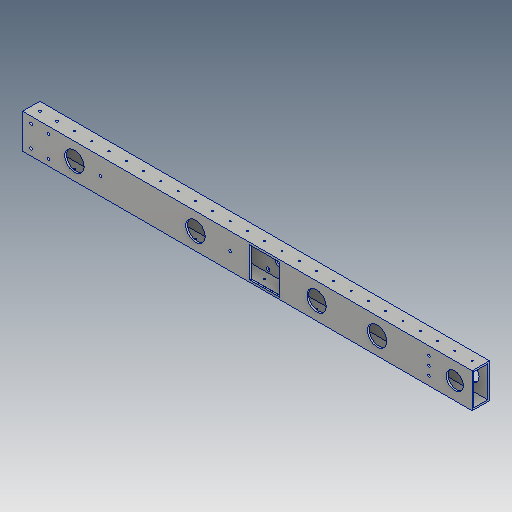
# Autodesk Inventor part: Vert Uprights
Saved by Autodesk Inventor 2018 (Build 220112000, 112)
## iProperties
Created: 2018-01-08
Part Number: Vert Uprights
Material: Aluminum 6061
Document SubType Name: Modeling
Designer: dsayers
Density: 2.7 g/cm^3
Appearance: Aluminum - Flat
Mass: 573.49 g
Surface Area: 1700.04 cm^2
Volume: 212.404 cm^3
Author: dsayers
Autodesk Inventor part; units mm, degrees
ref_plane "YZ Plane" through (0, 0, 0) normal (1, 0, 0) x (0, 1, 0)
ref_plane "XZ Plane" through (0, 0, 0) normal (0, 1, 0) x (-1, 0, 0)
ref_plane "XY Plane" through (0, 0, 0) normal (0, 0, 1) x (1, 0, 0)
sketch "Sketch1" plane through (0, 0, 0) normal (0, 0, 1) x (1, 0, 0)
  line L0 (0, 0) -> (25.4, 0)
  line L1 (25.4, 0) -> (25.4, 50.8)
  line L2 (25.4, 50.8) -> (0, 50.8)
  line L3 (0, 50.8) -> (0, 0)
  dimension "d0" = 25.4
  dimension "d1" = 50.8
  constraints: 8 end point, 2 parallel, 1 horizontal, 1 perpendicular
  measures "d0" distance of L1.end L2.end
  measures "d1" distance of L0.end L1.end
extrude "Extrusion1" add sketch "Sketch1" along normal blind 609.6
shell "Shell1" thickness 2.54 removed faces 2 at (8.4667, 33.8667, 0) at (8.4667, 33.8667, 609.6)
sketch "Sketch2" plane through (0, 50.8, 0) normal (0, 1, 0) x (1, 0, 0)
  line L0 (25.4, 0) -> (0, 0) projected
  line L1 (0, 0) -> (0, -609.6) projected
  point P0 (12.7, -12.7)
  point P1 (12.7, -38.1)
  point P2 (12.7, -63.5)
  point P3 (12.7, -88.9)
  point P4 (12.7, -114.3)
  point P5 (12.7, -139.7)
  point P6 (12.7, -165.1)
  point P7 (12.7, -190.5)
  point P8 (12.7, -215.9)
  point P9 (12.7, -241.3)
  point P10 (12.7, -266.7)
  point P11 (12.7, -292.1)
  point P12 (12.7, -317.5)
  point P13 (12.7, -342.9)
  point P14 (12.7, -368.3)
  point P15 (12.7, -393.7)
  point P16 (12.7, -419.1)
  point P17 (12.7, -444.5)
  point P18 (12.7, -469.9)
  point P19 (12.7, -495.3)
  point P20 (12.7, -520.7)
  point P21 (12.7, -546.1)
  point P22 (12.7, -571.5)
  point P23 (12.7, -596.9)
  point P24 (12.7, -622.3)
  point P25 (12.7, -647.7)
  point P26 (12.7, -673.1)
  point P27 (12.7, -698.5)
  point P28 (12.7, -723.9)
  point P29 (12.7, -749.3)
  point P30 (12.7, -774.7)
  point P31 (12.7, -800.1)
  point P32 (12.7, -825.5)
  point P33 (12.7, -850.9)
  point P34 (12.7, -876.3)
  point P35 (12.7, -901.7)
  point P36 (12.7, -927.1)
  dimension "d5" = 12.7
  dimension "d6" = 12.7
  dimension "d9" = 25.4
  constraints: 1 vertical, 36 other
  measures "d5" distance from line of L0 point (12.7, -12.7)
  measures "d6" distance from line of L1 point (12.7, -12.7)
  measures "d9" distance of point (12.7, -12.7) point (12.7, -38.1)
hole "Hole1" at (12.7, 50.8, 12.7) at (12.7, 50.8, 38.1) at (12.7, 50.8, 63.5) at (12.7, 50.8, 88.9) at (12.7, 50.8, 114.3) at (12.7, 50.8, 139.7) at (12.7, 50.8, 165.1) at (12.7, 50.8, 190.5) at (12.7, 50.8, 215.9) at (12.7, 50.8, 241.3) at (12.7, 50.8, 266.7) at (12.7, 50.8, 292.1) at (12.7, 50.8, 317.5) at (12.7, 50.8, 342.9) at (12.7, 50.8, 368.3) at (12.7, 50.8, 393.7) at (12.7, 50.8, 419.1) at (12.7, 50.8, 444.5) at (12.7, 50.8, 469.9) at (12.7, 50.8, 495.3) at (12.7, 50.8, 520.7) at (12.7, 50.8, 546.1) at (12.7, 50.8, 571.5) at (12.7, 50.8, 596.9) at (12.7, 50.8, 622.3) at (12.7, 50.8, 647.7) at (12.7, 50.8, 673.1) at (12.7, 50.8, 698.5) at (12.7, 50.8, 723.9) at (12.7, 50.8, 749.3) at (12.7, 50.8, 774.7) at (12.7, 50.8, 800.1) at (12.7, 50.8, 825.5) at (12.7, 50.8, 850.9) at (12.7, 50.8, 876.3) at (12.7, 50.8, 901.7) direction (0, -1, 0) diameter 2.54 depth 50.8 tip angle 118
sketch "Sketch6" plane through (0, 0, 0) normal (-1, 0, 0) x (0, 0, 1)
  line L0 (0, 50.8) -> (0, 0) projected
  line L1 (0, 0) -> (609.6, 0) projected
  point P0 (304.8, 25.4)
  dimension "d48" = 304.8
  dimension "d49" = 25.4
  measures "d48" distance from line of L0 point (304.8, 25.4)
  measures "d49" distance from line of L1 point (304.8, 25.4)
hole "Hole5" at (0, 25.4, 304.8) direction (1, 0, 0) diameter 15.875 depth 25.4 tip angle 118
sketch "Sketch7" plane through (25.4, 0, 0) normal (1, 0, 0) x (0, 0, -1)
  line L0 (0, 50.8) -> (-609.6, 50.8) projected
  circle A0 centre (-304.8, 25.4) radius 7.9375 projected
  point P0 (0, 0)
  point P1 (-584.2, 25.4)
  dimension "d57" = 25.4
  dimension "d58" = 279.4
  measures "d57" distance from line of L0 point (-584.2, 25.4)
  measures "d58" distance of A0.centre point (-584.2, 25.4)
hole "Hole6" at (25.4, 25.4, 584.2) direction (-1, 0, 0) diameter 25.4 depth 25.4 tip angle 118
sketch "Sketch8" plane through (0, 0, 0) normal (-1, 0, 0) x (0, 0, 1)
  circle A0 centre (304.8, 25.4) radius 7.9375 projected
  line L0 (282.575, 47.625) -> (327.025, 47.625)
  line L1 (327.025, 47.625) -> (327.025, 3.175)
  line L2 (327.025, 3.175) -> (282.575, 3.175)
  line L3 (282.575, 3.175) -> (282.575, 47.625)
  line L4 (282.575, 47.625) -> (327.025, 3.175) construction
  line L5 (327.025, 47.625) -> (282.575, 3.175) construction
  point P0 (0, 0)
  dimension "d66" = 44.45
  dimension "d67" = 44.45
  constraints: 12 end point, 2 midpoint, 2 parallel, 1 horizontal, 1 perpendicular
  measures "d66" distance of L0.end L1.end
  measures "d67" distance of L1.end L2.end
extrude "Extrusion2" cut sketch "Sketch8" against normal blind 12.7 contours A0 | L0 L1 L2 L3
sketch "Sketch9" plane through (25.4, 0, 0) normal (1, 0, 0) x (0, 0, -1)
  arc A0 (-320.6117, 44.0059) -> (-323.0807, 41.5866) centre (-322.5771, 43.5421) ccw projected
  arc A1 (-288.9883, 6.7941) -> (-286.5193, 9.2134) centre (-287.0229, 7.2579) ccw projected
  circle A2 centre (-322.4769, 8.0788) radius 3.3655 projected
  circle A3 centre (-287.1231, 42.7212) radius 3.1115 projected
  point P0 (0, 0)
  constraints: 4 coincident
hole "Hole7" at (25.4, 8.0788, 322.4769) at (25.4, 43.5421, 322.5771) at (25.4, 42.7212, 287.1231) at (25.4, 7.2579, 287.0229) direction (-1, 0, 0) diameter 5.6134 depth 25.4 tip angle 118 clearance for "Flat Head Machine Screw (82)" size "#10" standard "Ansi Unified Screw Threads"
sketch "Sketch10" plane through (0, 0, 0) normal (0, 0, -1) x (-1, 0, 0)
  line L0 (-2.54, 48.26) -> (-2.54, 2.54) projected
  line L1 (-2.54, 2.54) -> (-22.86, 2.54) projected
  line L2 (-22.86, 2.54) -> (-22.86, 48.26) projected
  line L3 (-22.86, 48.26) -> (-2.54, 48.26) projected
  line L4 (0, 0) -> (-25.4, 0) projected
  line L5 (0, 50.8) -> (0, 0) projected
  line L6 (-25.4, 50.8) -> (0, 50.8) projected
  line L7 (-25.4, 0) -> (-25.4, 50.8) projected
extrude "Extrusion3" add sketch "Sketch10" along normal blind 50.8
sketch "Sketch11" plane through (0, 50.8, 609.6) normal (0, 1, 0) x (1, 0, 0)
  circle A0 centre (12.7, 596.9) radius 1.27 projected
  line L0 (25.4, 660.4) -> (25.4, 0) projected
  point P0 (0, 609.6)
  point P1 (12.7, 622.3)
  point P2 (12.7, 647.7)
  dimension "d79" = 25.4
  dimension "d80" = 25.4
  dimension "d81" = 12.7
  dimension "d82" = 12.7
  measures "d79" distance of point (12.7, 622.3) point (12.7, 647.7)
  measures "d80" distance of A0.centre point (12.7, 622.3)
  measures "d81" distance from line of L0 point (12.7, 622.3)
  measures "d82" distance from line of L0 point (12.7, 647.7)
hole "Hole8" at (12.7, 50.8, -12.7) at (12.7, 50.8, -38.1) direction (0, -1, 0) diameter 3.9116 depth 50.8 tip angle 118 clearance for "Flat Head Machine Screw (82)" size "#5" standard "Ansi Unified Screw Threads"
sketch "Sketch12" plane through (0, 0, 609.6) normal (-1, 0, 0) x (0, 0, 1)
  circle A0 centre (-63.5, 25.4) radius 1.27 projected
  line L0 (0, 0) -> (-660.4, 0) projected
  line L1 (-660.4, 50.8) -> (0, 50.8) projected
  point P0 (-609.6, 0)
  point P1 (-63.5, 38.1)
  point P2 (-63.5, 12.7)
  dimension "d90" = 12.7
  dimension "d91" = 12.7
  dimension "d106" = 0
  dimension "d107" = 0
  constraints: 1 coincident
  measures "d90" distance from line of L0 point (-63.5, 12.7)
  measures "d91" distance from line of L1 point (-63.5, 38.1)
  measures "d106" horizontal distance of point (-63.5, 12.7) A0.centre
  measures "d107" horizontal distance of point (-63.5, 38.1) A0.centre
hole "Hole9" at (0, 25.4, 546.1) at (0, 38.1, 546.1) at (0, 12.7, 546.1) direction (1, 0, 0) diameter 3.9116 depth 50.8 tip angle 118 clearance for "Flat Head Machine Screw (82)" size "#5" standard "Ansi Unified Screw Threads"
sketch "Sketch13" plane through (0, 0, 609.6) normal (-1, 0, 0) x (0, 0, 1)
  circle A0 centre (-622.3, 533.4) radius 2.8067 projected
  circle A1 centre (-647.7, 533.4) radius 2.8067 projected
  circle A2 centre (-622.3, 584.2) radius 2.8067 projected
  circle A3 centre (-647.7, 584.2) radius 2.8067 projected
  circle A4 centre (-635, 558.8) radius 2.8067 projected
  circle A5 centre (-635, 190.5) radius 2.8067 projected
  circle A6 centre (-635, 762) radius 2.8067 projected
  circle A7 centre (-622.3, 762) radius 2.8067 projected
  circle A8 centre (-622.3, 558.8) radius 2.8067 projected
  circle A9 centre (-622.3, 190.5) radius 2.8067 projected
  circle A10 centre (-647.7, 190.5) radius 2.8067 projected
  circle A11 centre (-647.7, 558.8) radius 2.8067 projected
  circle A12 centre (-647.7, 762) radius 2.8067 projected
  circle A13 centre (-647.7, 41.275) radius 2.8067 projected
  circle A14 centre (-622.3, 41.275) radius 2.8067 projected
  circle A15 centre (-647.7, 9.525) radius 2.8067 projected
  circle A16 centre (-622.3, 9.525) radius 2.8067 projected
  circle A17 centre (-635, 374.65) radius 14.2875 projected
  circle A18 centre (-635, 114.3) radius 14.2875 projected
  circle A19 centre (-635, 730.25) radius 6.35 projected
  circle A20 centre (-635, 615.95) radius 6.35 projected
  circle A21 centre (-635, 649.2875) radius 2.8067 projected
  circle A22 centre (-635, 696.9125) radius 2.8067 projected
  circle A23 centre (-635, 673.1) radius 19.05 projected
  line L0 (-609.6, 774.7) -> (-660.4, 774.7) projected
  line L1 (-660.4, 774.7) -> (-660.4, -25.4) projected
  line L2 (-609.6, -25.4) -> (-660.4, -25.4) projected
  line L3 (-609.6, 774.7) -> (-609.6, -25.4) projected
  point P0 (-609.6, 0)
  constraints: 4 coincident
hole "Hole10" at (0, 41.275, -12.7) at (0, 9.525, -12.7) at (0, 9.525, -38.1) at (0, 41.275, -38.1) direction (1, 0, 0) diameter 3.9116 depth 50.8 tip angle 118 clearance for "Flat Head Machine Screw (82)" size "#5" standard "Ansi Unified Screw Threads"
sketch "Sketch14" plane through (0, 0, 609.6) normal (-1, 0, 0) x (0, 0, 1)
  circle A0 centre (-139.7, 25.4) radius 14.2875
  line L0 (-76.2, 546.1) -> (-76.2, 0) projected
  line L1 (0, 0) -> (-660.4, 0) projected
  point P0 (-609.6, 0)
  dimension "d108" = 63.5
  dimension "d109" = 28.575
  dimension "d110" = 25.4
  constraints: 1 centre point
  measures "d108" distance from line of L0 A0.centre
  measures "d109" diameter of A0
  measures "d110" distance from line of L1 A0.centre
extrude "Extrusion4" cut sketch "Sketch14" against normal blind 50.8
sketch "Sketch15" plane through (0, 0, 609.6) normal (-1, 0, 0) x (0, 0, 1)
  line L0 (0, 0) -> (-660.4, 0) projected
  line L1 (-660.4, 0) -> (-660.4, 50.8) projected
  point P0 (-609.6, 0)
  point P1 (-355.6, 25.4)
  dimension "d113" = 25.4
  dimension "d114" = 304.8
  measures "d113" distance from line of point (-355.6, 25.4) L0
  measures "d114" distance from line of L1 point (-355.6, 25.4)
hole "Hole11" at (0, 25.4, 254) direction (1, 0, 0) diameter 3.9116 depth 50.8 tip angle 118 clearance for "Flat Head Machine Screw (82)" size "#5" standard "Ansi Unified Screw Threads"
sketch "Sketch16" plane through (0, 0, 609.6) normal (-1, 0, 0) x (0, 0, 1)
  circle A0 centre (-546.1, 25.4) radius 1.27 projected
  point P0 (-609.6, 0)
  constraints: 1 coincident
hole "Hole12" at (0, 25.4, 63.5) direction (1, 0, 0) diameter 3.9116 depth 50.8 tip angle 118 clearance for "Flat Head Machine Screw (82)" size "#5" standard "Ansi Unified Screw Threads"
sketch "Sketch17" plane through (0, 0, 609.6) normal (-1, 0, 0) x (0, 0, 1)
  circle A0 centre (-584.2, 25.4) radius 14.2875
  line L0 (0, 0) -> (-660.4, 0) projected
  line L1 (-660.4, 0) -> (-660.4, 50.8) projected
  point P0 (-609.6, 0)
  dimension "d129" = 28.575
  dimension "d130" = 25.4
  dimension "d131" = 76.2
  constraints: 1 centre point
  measures "d129" diameter of A0
  measures "d130" distance from line of L0 A0.centre
  measures "d131" distance from line of L1 A0.centre
extrude "Extrusion5" cut sketch "Sketch17" against normal blind 50.8
sketch "Sketch18" plane through (0, 0, 609.6) normal (-1, 0, 0) x (0, 0, 1)
  circle A0 centre (-228.6, 25.4) radius 14.2875
  line L0 (0, 0) -> (-660.4, 0) projected
  circle A1 centre (-584.2, 25.4) radius 14.2875 projected
  point P0 (-609.6, 0)
  dimension "d134" = 28.575
  dimension "d135" = 25.4
  dimension "d136" = 355.6
  constraints: 1 centre point
  measures "d134" diameter of A0
  measures "d135" distance from line of L0 A0.centre
  measures "d136" distance of A1.centre A0.centre
extrude "Extrusion6" cut sketch "Sketch18" against normal blind 50.8 contours A0
sketch "Sketch19" plane through (0, 0, 609.6) normal (-1, 0, 0) x (0, 0, 1)
  circle A0 centre (-406.4, 25.4) radius 14.2875
  line L0 (0, 0) -> (-660.4, 0) projected
  circle A1 centre (-584.2, 25.4) radius 14.2875 projected
  point P0 (-609.6, 0)
  dimension "d139" = 25.4
  dimension "d140" = 177.8
  dimension "d141" = 28.575
  constraints: 1 centre point
  measures "d139" distance from line of L0 A0.centre
  measures "d140" distance of A1.centre A0.centre
  measures "d141" diameter of A0
extrude "Extrusion7" cut sketch "Sketch19" against normal blind 50.8 contours A0
equation "\"d67\" = d66"
body "Solid1"
